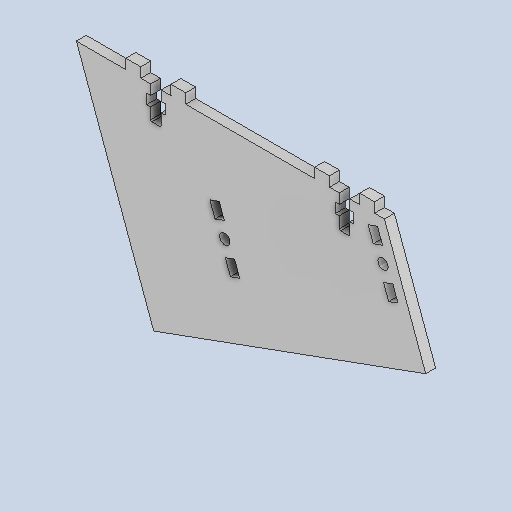
# Autodesk Inventor part: tc_support_front
Saved by Autodesk Inventor 2024.1 (Build 281209000, 209)
## iProperties
Created: 2019-07-16
Part Number: tc_support_front
Material: Générique
Document SubType Name: Modeling
Designer: Thibault
Density: 1 g/cm^3
Appearance: Par défaut
Author: Thibault
Autodesk Inventor part; units mm, degrees
ref_plane "YZ Plane" through (0, 0, 0) normal (1, 0, 0) x (0, 1, 0)
ref_plane "XZ Plane" through (0, 0, 0) normal (0, 1, 0) x (-1, 0, 0)
ref_plane "XY Plane" through (0, 0, 0) normal (0, 0, 1) x (1, 0, 0)
sketch "Anchor (nut side)" plane through (0, 0, 0) normal (0, 0, 1) x (1, 0, 0)
  line L0 (11.1, 0) -> (9.1, 0)
  line L1 (9.1, 0) -> (9.1, -2)
  line L2 (9.1, -2) -> (9.9, -2)
  line L3 (9.9, -2) -> (9.9, -4)
  line L4 (6.2, -4) -> (6.2, -2)
  line L5 (6.2, -2) -> (7, -2)
  line L6 (7, -2) -> (7, 0)
  line L7 (7, 0) -> (5, 0)
  line L8 (2, 0) -> (2, 2)
  line L9 (2, 0) -> (3, 0) construction
  line L10 (2, 2) -> (5, 2)
  line L11 (5, 2) -> (5, 0)
  line L12 (11.1, 0) -> (11.1, 2)
  line L13 (11.1, 2) -> (14.1, 2)
  line L14 (14.1, 2) -> (14.1, 0)
  line L15 (0, 0) -> (2, 0)
  line L16 (14.1, 0) -> (16.1, 0)
  line L17 (6.2, -4) -> (7, -4)
  line L18 (9.9, -4) -> (9.1, -4)
  line L19 (7, -4) -> (7, -6.25)
  line L20 (9.1, -4) -> (9.1, -6.25)
  line L21 (7.25, -6.5) -> (8.05, -6.5)
  arc A0 (7, -6.25) -> (7.25, -6.5) centre (7.25, -6.25) ccw
  arc A1 (8.85, -6.5) -> (9.1, -6.25) centre (8.85, -6.25) ccw
  line L22 (8.05, -6.5) -> (8.85, -6.5)
  line L23 (8.05, -3.8983) -> (8.05, -9.959) construction
  point P0 (9.1321, -0.6227)
  point P1 (7, -6.5)
  point P2 (9.1, -6.5)
  dimension "d3" = 2
  dimension "d7" = 6.1
  dimension "d10" = 2
  dimension "d11" = 2
  dimension "d12" = 0.8
  dimension "d13" = 2
  dimension "d14" = 0.8
  dimension "d15" = 2.1
  dimension "d18" = 2
  dimension "d19" = 0.8
  dimension "d20" = 0.8
  dimension "d21" = 2.5
  dimension "d22" = 2.5
  dimension "d23" = 2.1
  dimension "d38" = 2
  dimension "d39" = 0.25
  dimension "d120" = 3
  measures "d3" distance of L15.start L8.start
  measures "d7" distance of L7.end L0.start
  measures "d10" distance of L0.start L0.end
  measures "d11" distance of L0.end L1.end
  measures "d12" distance of L1.end L2.end
  measures "d13" distance of L2.end L3.end
  measures "d14" distance of L4.end L5.end
  measures "d15" distance of L6.end L0.end
  measures "d18" distance of L14.end L16.end
  measures "d19" distance of L4.start L17.end
  measures "d20" distance of L3.end L18.end
  measures "d21" distance of L17.end point (7, -6.5)
  measures "d22" distance of L18.end point (9.1, -6.5)
  measures "d23" distance of L17.end L18.end
  measures "d38" distance between parallel lines of L15 L10
  measures "d39" radius of A0
  measures "d120" distance of L8.end L10.end
sketch "Anchor (screw side)" plane through (0, 0, 0) normal (0, 0, 1) x (1, 0, 0)
  circle A0 centre (93.8994, 50.2542) radius 1.05
  line L0 (90.8494, 51.2542) -> (87.8494, 51.2542)
  line L1 (87.8494, 51.2542) -> (87.8494, 49.2542)
  line L2 (87.8494, 49.2542) -> (90.8494, 49.2542)
  line L3 (90.8494, 49.2542) -> (90.8494, 51.2542)
  line L4 (99.9494, 51.2542) -> (96.9494, 51.2542)
  line L5 (96.9494, 51.2542) -> (96.9494, 49.2542)
  line L6 (96.9494, 49.2542) -> (99.9494, 49.2542)
  line L7 (99.9494, 49.2542) -> (99.9494, 51.2542)
  line L8 (90.8494, 51.2542) -> (96.9494, 49.2542) construction
  line L9 (96.9494, 51.2542) -> (90.8494, 49.2542) construction
  line L10 (85.8494, 53.2542) -> (101.9494, 53.2542) construction
  line L11 (101.9494, 53.2542) -> (101.9494, 47.2542) construction
  line L12 (101.9494, 47.2542) -> (85.8494, 47.2542) construction
  line L13 (85.8494, 47.2542) -> (85.8494, 53.2542) construction
  point P0 (103.5798, 50.1132)
  dimension "d27" = 2.1
  dimension "d28" = 3
  dimension "d29" = 2
  dimension "slot_distance" = 6.1
  dimension "d34" = 2
  dimension "d35_1" = 2
  dimension "d36_1" = 2
  dimension "d37" = 2
  measures "d27" diameter of A0
  measures "d28" distance of L2.end L1.end
  measures "d29" distance of L1.end L0.end
  measures "slot_distance" distance between parallel lines of L5 L3
  measures "d34" distance between parallel lines of L0 L10
  measures "d35_1" distance between parallel lines of L12 L2
  measures "d36_1" distance between parallel lines of L11 L7
  measures "d37" distance between parallel lines of L13 L1
derived "shared_parameters.ipt"
sketch "Esquisse1" plane through (0, 0, 0) normal (0, 0, 1) x (1, 0, 0)
  line L0 (-6.4537, 6.9042) -> (15.5463, 6.9042)
  line L1 (-22.5537, 6.9042) -> (-30.5537, 6.9042)
  line L2 (39.9818, -15.9975) -> (31.6463, 6.9042)
  line L3 (39.9818, -15.9975) -> (-14.9421, -35.9882)
  line L4 (-2.0657, -1.8526) -> (7.9343, -1.7975) construction
  line L5 (-14.9421, -35.9882) -> (-30.5537, 6.9042)
  line L6 (-11.4537, 6.9042) -> (-13.4537, 6.9042)
  line L7 (-13.4537, 6.9042) -> (-13.4537, 4.9042)
  line L8 (-13.4537, 4.9042) -> (-12.6537, 4.9042)
  line L9 (-12.6537, 4.9042) -> (-12.6537, 2.9042)
  line L10 (-16.3537, 2.9042) -> (-16.3537, 4.9042)
  line L11 (-16.3537, 4.9042) -> (-15.5537, 4.9042)
  line L12 (-15.5537, 4.9042) -> (-15.5537, 6.9042)
  line L13 (-15.5537, 6.9042) -> (-17.5537, 6.9042)
  line L14 (-20.5537, 6.9042) -> (-20.5537, 8.9042)
  line L15 (-20.5537, 6.9042) -> (-19.5537, 6.9042) construction
  line L16 (-20.5537, 8.9042) -> (-17.5537, 8.9042)
  line L17 (-17.5537, 8.9042) -> (-17.5537, 6.9042)
  line L18 (-11.4537, 6.9042) -> (-11.4537, 8.9042)
  line L19 (-11.4537, 8.9042) -> (-8.4537, 8.9042)
  line L20 (-8.4537, 8.9042) -> (-8.4537, 6.9042)
  line L21 (-22.5537, 6.9042) -> (-20.5537, 6.9042)
  line L22 (-8.4537, 6.9042) -> (-6.4537, 6.9042)
  line L23 (-16.3537, 2.9042) -> (-15.5537, 2.9042)
  line L24 (-12.6537, 2.9042) -> (-13.4537, 2.9042)
  line L25 (-15.5537, 2.9042) -> (-15.5537, 0.6542)
  line L26 (-13.4537, 2.9042) -> (-13.4537, 0.6542)
  line L27 (-15.3037, 0.4042) -> (-14.5037, 0.4042)
  arc A0 (-15.5537, 0.6542) -> (-15.3037, 0.4042) centre (-15.3037, 0.6542) ccw
  arc A1 (-13.7037, 0.4042) -> (-13.4537, 0.6542) centre (-13.7037, 0.6542) ccw
  line L28 (-14.5037, 0.4042) -> (-13.7037, 0.4042)
  line L29 (-14.5037, 3.006) -> (-14.5037, -3.0548) construction
  line L30 (26.6463, 6.9042) -> (24.6463, 6.9042)
  line L31 (24.6463, 6.9042) -> (24.6463, 4.9042)
  line L32 (24.6463, 4.9042) -> (25.4463, 4.9042)
  line L33 (25.4463, 4.9042) -> (25.4463, 2.9042)
  line L34 (21.7463, 2.9042) -> (21.7463, 4.9042)
  line L35 (21.7463, 4.9042) -> (22.5463, 4.9042)
  line L36 (22.5463, 4.9042) -> (22.5463, 6.9042)
  line L37 (22.5463, 6.9042) -> (20.5463, 6.9042)
  line L38 (17.5463, 6.9042) -> (17.5463, 8.9042)
  line L39 (17.5463, 6.9042) -> (18.5463, 6.9042) construction
  line L40 (17.5463, 8.9042) -> (20.5463, 8.9042)
  line L41 (20.5463, 8.9042) -> (20.5463, 6.9042)
  line L42 (26.6463, 6.9042) -> (26.6463, 8.9042)
  line L43 (26.6463, 8.9042) -> (29.6463, 8.9042)
  line L44 (29.6463, 8.9042) -> (29.6463, 6.9042)
  line L45 (15.5463, 6.9042) -> (17.5463, 6.9042)
  line L46 (29.6463, 6.9042) -> (31.6463, 6.9042)
  line L47 (21.7463, 2.9042) -> (22.5463, 2.9042)
  line L48 (25.4463, 2.9042) -> (24.6463, 2.9042)
  line L49 (22.5463, 2.9042) -> (22.5463, 0.6542)
  line L50 (24.6463, 2.9042) -> (24.6463, 0.6542)
  line L51 (22.7963, 0.4042) -> (23.5963, 0.4042)
  arc A2 (22.5463, 0.6542) -> (22.7963, 0.4042) centre (22.7963, 0.6542) ccw
  arc A3 (24.3963, 0.4042) -> (24.6463, 0.6542) centre (24.3963, 0.6542) ccw
  line L52 (23.5963, 0.4042) -> (24.3963, 0.4042)
  line L53 (23.5963, 3.006) -> (23.5963, -3.0548) construction
  circle A4 centre (31.3655, -1.0958) radius 1.05
  line L54 (31.469, -4.3038) -> (32.4951, -7.1229)
  line L55 (32.4951, -7.1229) -> (34.3744, -6.4389)
  line L56 (34.3744, -6.4389) -> (33.3484, -3.6198)
  line L57 (33.3484, -3.6198) -> (31.469, -4.3038)
  line L58 (28.3566, 4.2474) -> (29.3827, 1.4283)
  line L59 (29.3827, 1.4283) -> (31.2621, 2.1123)
  line L60 (31.2621, 2.1123) -> (30.236, 4.9314)
  line L61 (30.236, 4.9314) -> (28.3566, 4.2474)
  line L62 (31.469, -4.3038) -> (31.2621, 2.1123) construction
  line L63 (29.3827, 1.4283) -> (33.3484, -3.6198) construction
  line L64 (31.2997, -9.6863) -> (25.7932, 5.4427) construction
  line L65 (25.7932, 5.4427) -> (31.4313, 7.4948) construction
  line L66 (31.4313, 7.4948) -> (36.9379, -7.6342) construction
  line L67 (36.9379, -7.6342) -> (31.2997, -9.6863) construction
  circle A5 centre (-0.584, -12.7244) radius 1.05
  line L68 (-0.6875, -9.5164) -> (-1.7136, -6.6973)
  line L69 (-1.7136, -6.6973) -> (-3.5929, -7.3813)
  line L70 (-3.5929, -7.3813) -> (-2.5669, -10.2004)
  line L71 (-2.5669, -10.2004) -> (-0.6875, -9.5164)
  line L72 (2.4249, -18.0676) -> (1.3988, -15.2485)
  line L73 (1.3988, -15.2485) -> (-0.4806, -15.9325)
  line L74 (-0.4806, -15.9325) -> (0.5455, -18.7516)
  line L75 (0.5455, -18.7516) -> (2.4249, -18.0676)
  line L76 (-0.6875, -9.5164) -> (-0.4806, -15.9325) construction
  line L77 (1.3988, -15.2485) -> (-2.5669, -10.2004) construction
  line L78 (-0.5182, -4.1339) -> (4.9883, -19.2629) construction
  line L79 (4.9883, -19.2629) -> (-0.6498, -21.315) construction
  line L80 (-0.6498, -21.315) -> (-6.1564, -6.186) construction
  line L81 (-6.1564, -6.186) -> (-0.5182, -4.1339) construction
  point P0 (22.4992, -2.0098)
  point P1 (31.3655, -1.0958)
  point P2 (-0.584, -12.7244)
  point P3 (31.6463, 6.9042)
  dimension "d33" = 62.2
  dimension "d44" = 10.9
  dimension "d49" = 10
  dimension "d52" = 2
  dimension "d53" = 36
  dimension "d54" = 8
  dimension "d58" = 20
  constraints: 12 end point, 3 horizontal, 1 parallel, 1 perpendicular, 6 other
  measures "d33" distance of L1.end L2.end
  measures "d58" angle of L3 L0
extrude "Extrusion1" add sketch "Esquisse1" along normal blind 2
derived "tc_base_plate.ipt"
equation "\"d33\" = tc_base_width"
equation "\"d44\" = extra_height_front"
equation "\"d52\" = anchor_dist_a"
equation "\"d53\" = anchor_dist_b"
equation "\"d54\" = anchor_dist_top_a"
equation "\"d58\" = tilt_angle"
equation "\"d35\" = sheet_thickness"
equation "\"tc_base_width\" = 62.2"
equation "\"extra_height_front\" = 10.9"
equation "\"anchor_dist_a\" = 2"
equation "\"anchor_dist_b\" = 36"
equation "\"anchor_dist_top_a\" = 8"
equation "\"tilt_angle\" = 20deg"
equation "\"sheet_thickness\" = 2"
